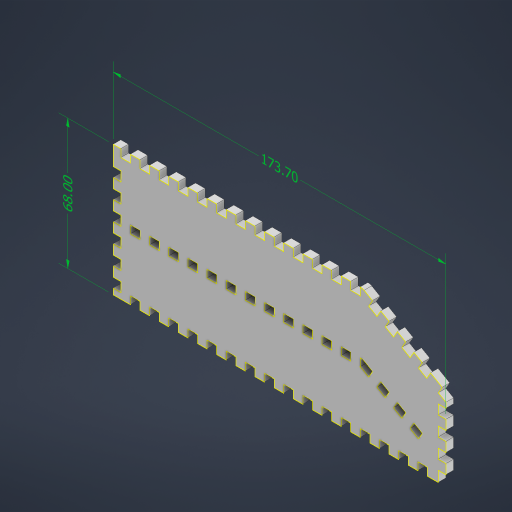
# Autodesk Inventor part: SeitenWand
Saved by Autodesk Inventor 2023 (Build 270158030, 158C)
## iProperties
Created: 2022-06-21
Part Number: SeitenWand
Material: Generic
Document SubType Name: Modeling
Designer: Simon
Density: 1 g/cm^3
Appearance: Default
Author: Simon
Autodesk Inventor part; units mm, degrees
ref_plane "YZ Plane" through (0, 0, 0) normal (1, 0, 0) x (0, 1, 0)
ref_plane "XZ Plane" through (0, 0, 0) normal (0, 1, 0) x (-1, 0, 0)
ref_plane "XY Plane" through (0, 0, 0) normal (0, 0, 1) x (1, 0, 0)
sketch "Sketch1" plane through (0, 0, 0) normal (0, 0, 1) x (1, 0, 0)
  line L0 (86, 30) -> (-86, 30)
  line L1 (-86, 30) -> (-86, -30)
  line L2 (-86, -30) -> (86, -30)
  line L3 (86, -30) -> (86, 30)
  line L4 (86, 30) -> (-86, -30) construction
  line L5 (-86, 30) -> (86, -30) construction
  line L6 (39, 30) -> (79.7032, 6.5)
  line L7 (39, 30) -> (86, 30) construction
  line L8 (79.7032, 6.5) -> (79.7032, -30)
  circle A0 centre (39, 30) radius 47
  point P0 (0, 0)
  dimension "d0" = 172
  dimension "d1" = 60
  dimension "d2" = 47
  dimension "d3" = 30
  dimension "d4" = 125
  constraints: 18 end point, 2 horizontal, 2 midpoint, 2 parallel, 2 perpendicular, 2 point on line, 1 coincident, 1 equal length, 3 other
  measures "d0" distance of L2.end L1.end
  measures "d1" distance of L1.end L0.end
  measures "d2" distance of L6.start L6.end
  measures "d3" angle of L6 L7
  measures "d4" distance of L0.end L6.start
extrude "Extrusion1" add sketch "Sketch1" along normal blind 4 contours L6 A0 L0 | L8 L2 L1 L0 A0 picked at (64.2944, 11.7777)
sketch "Sketch2" plane through (0, 0, 4) normal (0, 0, 1) x (1, 0, 0)
  line L0 (39, 30) -> (-86, 30) projected
  line L1 (-81, 30) -> (-76, 30)
  line L2 (-76, 30) -> (-76, 34)
  line L3 (-76, 34) -> (-81, 34)
  line L4 (-81, 34) -> (-81, 30)
  line L5 (-71, 30) -> (-66, 30)
  line L6 (-66, 30) -> (-66, 34)
  line L7 (-66, 34) -> (-71, 34)
  line L8 (-71, 34) -> (-71, 30)
  line L9 (-61, 30) -> (-56, 30)
  line L10 (-56, 30) -> (-56, 34)
  line L11 (-56, 34) -> (-61, 34)
  line L12 (-61, 34) -> (-61, 30)
  line L13 (-51, 30) -> (-46, 30)
  line L14 (-46, 30) -> (-46, 34)
  line L15 (-46, 34) -> (-51, 34)
  line L16 (-51, 34) -> (-51, 30)
  line L17 (-41, 30) -> (-36, 30)
  line L18 (-36, 30) -> (-36, 34)
  line L19 (-36, 34) -> (-41, 34)
  line L20 (-41, 34) -> (-41, 30)
  line L21 (-31, 30) -> (-26, 30)
  line L22 (-26, 30) -> (-26, 34)
  line L23 (-26, 34) -> (-31, 34)
  line L24 (-31, 34) -> (-31, 30)
  line L25 (-21, 30) -> (-16, 30)
  line L26 (-16, 30) -> (-16, 34)
  line L27 (-16, 34) -> (-21, 34)
  line L28 (-21, 34) -> (-21, 30)
  line L29 (-11, 30) -> (-6, 30)
  line L30 (-6, 30) -> (-6, 34)
  line L31 (-6, 34) -> (-11, 34)
  line L32 (-11, 34) -> (-11, 30)
  line L33 (-1, 30) -> (4, 30)
  line L34 (4, 30) -> (4, 34)
  line L35 (4, 34) -> (-1, 34)
  line L36 (-1, 34) -> (-1, 30)
  line L37 (9, 30) -> (14, 30)
  line L38 (14, 30) -> (14, 34)
  line L39 (14, 34) -> (9, 34)
  line L40 (9, 34) -> (9, 30)
  line L41 (19, 30) -> (24, 30)
  line L42 (24, 30) -> (24, 34)
  line L43 (24, 34) -> (19, 34)
  line L44 (19, 34) -> (19, 30)
  line L45 (29, 30) -> (34, 30)
  line L46 (34, 30) -> (34, 34)
  line L47 (34, 34) -> (29, 34)
  line L48 (29, 34) -> (29, 30)
  line L49 (79.7032, 6.5) -> (39, 30) projected
  line L50 (39, 30) -> (43.3301, 27.5)
  line L51 (43.3301, 27.5) -> (45.3301, 30.9641)
  line L52 (45.3301, 30.9641) -> (41, 33.4641)
  line L53 (41, 33.4641) -> (39, 30)
  line L54 (39, 30) -> (39, 34)
  arc A0 (41, 33.4641) -> (39, 34) centre (39, 30) ccw
  line L55 (53.9904, 25.9641) -> (49.6603, 28.4641)
  line L56 (49.6603, 28.4641) -> (47.6603, 25)
  line L57 (51.9904, 22.5) -> (53.9904, 25.9641)
  line L58 (47.6603, 25) -> (51.9904, 22.5)
  line L59 (62.6506, 20.9641) -> (58.3205, 23.4641)
  line L60 (58.3205, 23.4641) -> (56.3205, 20)
  line L61 (60.6506, 17.5) -> (62.6506, 20.9641)
  line L62 (56.3205, 20) -> (60.6506, 17.5)
  line L63 (71.3109, 15.9641) -> (66.9808, 18.4641)
  line L64 (66.9808, 18.4641) -> (64.9808, 15)
  line L65 (69.3109, 12.5) -> (71.3109, 15.9641)
  line L66 (64.9808, 15) -> (69.3109, 12.5)
  line L67 (79.9711, 10.9641) -> (75.641, 13.4641)
  line L68 (75.641, 13.4641) -> (73.641, 10)
  line L69 (77.9711, 7.5) -> (79.9711, 10.9641)
  line L70 (73.641, 10) -> (77.9711, 7.5)
  line L71 (75.641, 13.4641) -> (81.7032, 9.9641)
  line L72 (81.7032, 9.9641) -> (79.7032, 6.5)
  line L73 (-81, -2) -> (-76, -2)
  line L74 (-76, -2) -> (-76, 2)
  line L75 (-76, 2) -> (-81, 2)
  line L76 (-81, 2) -> (-81, -2)
  line L77 (-81, -2) -> (-76, 2) construction
  line L78 (-76, -2) -> (-81, 2) construction
  line L79 (-66, -2) -> (-66, 2)
  line L80 (-66, 2) -> (-71, 2)
  line L81 (-71, -2) -> (-66, -2)
  line L82 (-71, 2) -> (-71, -2)
  line L83 (-71, -2) -> (-66, 2) construction
  line L84 (-66, -2) -> (-71, 2) construction
  line L85 (-56, -2) -> (-56, 2)
  line L86 (-56, 2) -> (-61, 2)
  line L87 (-61, -2) -> (-56, -2)
  line L88 (-61, 2) -> (-61, -2)
  line L89 (-61, -2) -> (-56, 2) construction
  line L90 (-56, -2) -> (-61, 2) construction
  line L91 (-46, -2) -> (-46, 2)
  line L92 (-46, 2) -> (-51, 2)
  line L93 (-51, -2) -> (-46, -2)
  line L94 (-51, 2) -> (-51, -2)
  line L95 (-51, -2) -> (-46, 2) construction
  line L96 (-46, -2) -> (-51, 2) construction
  line L97 (-36, -2) -> (-36, 2)
  line L98 (-36, 2) -> (-41, 2)
  line L99 (-41, -2) -> (-36, -2)
  line L100 (-41, 2) -> (-41, -2)
  line L101 (-41, -2) -> (-36, 2) construction
  line L102 (-36, -2) -> (-41, 2) construction
  line L103 (-26, -2) -> (-26, 2)
  line L104 (-26, 2) -> (-31, 2)
  line L105 (-31, -2) -> (-26, -2)
  line L106 (-31, 2) -> (-31, -2)
  line L107 (-31, -2) -> (-26, 2) construction
  line L108 (-26, -2) -> (-31, 2) construction
  line L109 (-16, -2) -> (-16, 2)
  line L110 (-16, 2) -> (-21, 2)
  line L111 (-21, -2) -> (-16, -2)
  line L112 (-21, 2) -> (-21, -2)
  line L113 (-21, -2) -> (-16, 2) construction
  line L114 (-16, -2) -> (-21, 2) construction
  line L115 (-6, -2) -> (-6, 2)
  line L116 (-6, 2) -> (-11, 2)
  line L117 (-11, -2) -> (-6, -2)
  line L118 (-11, 2) -> (-11, -2)
  line L119 (-11, -2) -> (-6, 2) construction
  line L120 (-6, -2) -> (-11, 2) construction
  line L121 (4, -2) -> (4, 2)
  line L122 (4, 2) -> (-1, 2)
  line L123 (-1, -2) -> (4, -2)
  line L124 (-1, 2) -> (-1, -2)
  line L125 (-1, -2) -> (4, 2) construction
  line L126 (4, -2) -> (-1, 2) construction
  line L127 (14, -2) -> (14, 2)
  line L128 (14, 2) -> (9, 2)
  line L129 (9, -2) -> (14, -2)
  line L130 (9, 2) -> (9, -2)
  line L131 (9, -2) -> (14, 2) construction
  line L132 (14, -2) -> (9, 2) construction
  line L133 (24, -2) -> (24, 2)
  line L134 (24, 2) -> (19, 2)
  line L135 (19, -2) -> (24, -2)
  line L136 (19, 2) -> (19, -2)
  line L137 (19, -2) -> (24, 2) construction
  line L138 (24, -2) -> (19, 2) construction
  line L139 (34, -2) -> (34, 2)
  line L140 (34, 2) -> (29, 2)
  line L141 (29, -2) -> (34, -2)
  line L142 (29, 2) -> (29, -2)
  line L143 (29, -2) -> (34, 2) construction
  line L144 (34, -2) -> (29, 2) construction
  line L145 (39, -2) -> (43.3301, -4.5)
  line L146 (43.3301, -4.5) -> (45.3301, -1.0359)
  line L147 (45.3301, -1.0359) -> (41, 1.4641)
  line L148 (41, 1.4641) -> (39, -2)
  line L149 (39, -2) -> (44, -2) construction
  line L150 (39, -2) -> (39, 2)
  arc A1 (41, 1.4641) -> (39, 2) centre (39, -2) ccw
  line L151 (51.9904, -9.5) -> (53.9904, -6.0359)
  line L152 (47.6603, -7) -> (51.9904, -9.5)
  line L153 (49.6603, -3.5359) -> (47.6603, -7)
  line L154 (53.9904, -6.0359) -> (49.6603, -3.5359)
  line L155 (60.6506, -14.5) -> (62.6506, -11.0359)
  line L156 (56.3205, -12) -> (60.6506, -14.5)
  line L157 (58.3205, -8.5359) -> (56.3205, -12)
  line L158 (62.6506, -11.0359) -> (58.3205, -8.5359)
  line L159 (69.3109, -19.5) -> (71.3109, -16.0359)
  line L160 (64.9808, -17) -> (69.3109, -19.5)
  line L161 (66.9808, -13.5359) -> (64.9808, -17)
  line L162 (71.3109, -16.0359) -> (66.9808, -13.5359)
  line L163 (-86, -30) -> (79.7032, -30) projected
  line L164 (-86, -30) -> (-81, -30)
  line L165 (-81, -30) -> (-81, -34)
  line L166 (-81, -34) -> (-86, -34)
  line L167 (-86, -34) -> (-86, -30)
  line L168 (-71, -30) -> (-71, -34)
  line L169 (-76, -30) -> (-71, -30)
  line L170 (-76, -34) -> (-76, -30)
  line L171 (-71, -34) -> (-76, -34)
  line L172 (-61, -30) -> (-61, -34)
  line L173 (-66, -30) -> (-61, -30)
  line L174 (-66, -34) -> (-66, -30)
  line L175 (-61, -34) -> (-66, -34)
  line L176 (-51, -30) -> (-51, -34)
  line L177 (-56, -30) -> (-51, -30)
  line L178 (-56, -34) -> (-56, -30)
  line L179 (-51, -34) -> (-56, -34)
  line L180 (-41, -30) -> (-41, -34)
  line L181 (-46, -30) -> (-41, -30)
  line L182 (-46, -34) -> (-46, -30)
  line L183 (-41, -34) -> (-46, -34)
  line L184 (-31, -30) -> (-31, -34)
  line L185 (-36, -30) -> (-31, -30)
  line L186 (-36, -34) -> (-36, -30)
  line L187 (-31, -34) -> (-36, -34)
  line L188 (-21, -30) -> (-21, -34)
  line L189 (-26, -30) -> (-21, -30)
  line L190 (-26, -34) -> (-26, -30)
  line L191 (-21, -34) -> (-26, -34)
  line L192 (-11, -30) -> (-11, -34)
  line L193 (-16, -30) -> (-11, -30)
  line L194 (-16, -34) -> (-16, -30)
  line L195 (-11, -34) -> (-16, -34)
  line L196 (-1, -30) -> (-1, -34)
  line L197 (-6, -30) -> (-1, -30)
  line L198 (-6, -34) -> (-6, -30)
  line L199 (-1, -34) -> (-6, -34)
  line L200 (9, -30) -> (9, -34)
  line L201 (4, -30) -> (9, -30)
  line L202 (4, -34) -> (4, -30)
  line L203 (9, -34) -> (4, -34)
  line L204 (19, -30) -> (19, -34)
  line L205 (14, -30) -> (19, -30)
  line L206 (14, -34) -> (14, -30)
  line L207 (19, -34) -> (14, -34)
  line L208 (29, -30) -> (29, -34)
  line L209 (24, -30) -> (29, -30)
  line L210 (24, -34) -> (24, -30)
  line L211 (29, -34) -> (24, -34)
  line L212 (39, -30) -> (39, -34)
  line L213 (34, -30) -> (39, -30)
  line L214 (34, -34) -> (34, -30)
  line L215 (39, -34) -> (34, -34)
  line L216 (49, -30) -> (49, -34)
  line L217 (44, -30) -> (49, -30)
  line L218 (44, -34) -> (44, -30)
  line L219 (49, -34) -> (44, -34)
  line L220 (59, -30) -> (59, -34)
  line L221 (54, -30) -> (59, -30)
  line L222 (54, -34) -> (54, -30)
  line L223 (59, -34) -> (54, -34)
  line L224 (69, -30) -> (69, -34)
  line L225 (64, -30) -> (69, -30)
  line L226 (64, -34) -> (64, -30)
  line L227 (69, -34) -> (64, -34)
  line L228 (79, -30) -> (79, -34)
  line L229 (74, -30) -> (79, -30)
  line L230 (74, -34) -> (74, -30)
  line L231 (79, -34) -> (74, -34)
  line L232 (79.7032, -30) -> (79, -30)
  line L233 (79, -30) -> (79, -34)
  line L234 (79, -34) -> (79.7032, -34)
  line L235 (79.7032, -34) -> (79.7032, -30)
  point P0 (0, 0)
  point P1 (-78.5, 0)
  point P2 (-68.5, 0)
  point P3 (-58.5, 0)
  point P4 (-48.5, 0)
  point P5 (-38.5, 0)
  point P6 (-28.5, 0)
  point P7 (-18.5, 0)
  point P8 (-8.5, 0)
  point P9 (1.5, 0)
  point P10 (11.5, 0)
  point P11 (21.5, 0)
  point P12 (31.5, 0)
  dimension "d7" = 5
  dimension "d8" = 4
  dimension "d11" = 10
  dimension "d16" = 5
  dimension "d17" = 4
  dimension "d20" = 10
  dimension "d25" = 7
  dimension "d26" = 5
  dimension "d27" = 4
  dimension "d30" = 10
  dimension "d35" = 5
  dimension "d36" = 30
  dimension "d37" = 4
  dimension "d40" = 10
  dimension "d45" = 5
  dimension "d46" = 4
  dimension "d49" = 10
  constraints: 466 end point, 108 horizontal alignment, 66 parallel, 57 collinear, 6 horizontal, 6 perpendicular, 4 point on circle, 4 point on line, 2 centre point, 2 midpoint, 2 tangent, 2 vertical, 1 equal length, 179 other
  measures "d7" distance of L3.end L2.end
  measures "d8" distance of L2.end L1.end
  measures "d11" distance of L1.start L5.start
  measures "d16" distance of L49.end L50.end
  measures "d17" distance of L51.end L50.end
  measures "d20" distance of L51.end L55.start
  measures "d25" distance of L67.end L71.end
  measures "d26" distance of L75.end L74.end
  measures "d27" distance of L74.end L73.end
  measures "d30" distance of L73.end L79.start
  measures "d35" distance of L145.start L145.end
  measures "d36" angle of L145 L149
  measures "d37" distance of L146.end L145.end
  measures "d40" distance of L145.end L151.start
  measures "d45" distance of L165.end L166.end
  measures "d46" distance of L164.end L165.end
  measures "d49" distance of L164.end L168.start
extrude "Extrusion2" add sketch "Sketch2" against normal blind 4 contours L0 L48 L47 L46 | L0 L44 L43 L42 | L0 L40 L39 L38 | L0 L36 L35 L34 | L0 L32 L31 L30 | L0 L28 L27 L26 | L0 L24 L23 L22 | L0 L20 L19 L18 | L0 L16 L15 L14 | L0 L12 L11 L10 | L0 L8 L7 L6 | L0 L4 L3 L2 | L49 L69 L71 L72 | L49 L68 L67 L69 | L49 L64 L63 L65 | L49 L60 L59 L61 | L49 L56 L55 L57 | L49 L53 L52 L51 | L54 A0 L53 | L163 L165 L166 L167 | L163 L168 L171 L170 | L163 L172 L175 L174 | L163 L176 L179 L178 | L163 L180 L183 L182 | L163 L184 L187 L186 | L163 L188 L191 L190 | L163 L192 L195 L194 | L163 L196 L199 L198 | L163 L200 L203 L202 | L163 L204 L207 L206 | L163 L208 L211 L210 | L163 L212 L215 L214 | L163 L216 L219 L218 | L163 L220 L223 L222 | L163 L224 L227 L226 | L163 L228 L231 L230 | L163 L235 L234 L228
extrude "Extrusion3" cut sketch "Sketch2" against normal blind 4 contours L76 L75 L74 L73 | L81 L82 L80 L79 | L87 L88 L86 L85 | L93 L94 L92 L91 | L99 L100 L98 L97 | L105 L106 L104 L103 | L111 L112 L110 L109 | L117 L118 L116 L115 | L123 L124 L122 L121 | L129 L130 L128 L127 | L135 L136 L134 L133 | L141 L142 L140 L139 | L148 L147 L146 L145 | L150 A1 L148 | L152 L153 L154 L151 | L156 L157 L158 L155 | L160 L161 L162 L159
sketch "Sketch3" plane through (0, 0, 4) normal (0, 0, 1) x (1, 0, 0)
  line L0 (-86, 34) -> (-90, 34)
  line L1 (-90, 34) -> (-90, 24)
  line L2 (-90, 24) -> (-86, 24)
  line L3 (-86, 24) -> (-86, 34)
  line L4 (-86, 30) -> (-86, -34) projected
  line L5 (-86, 19) -> (-90, 19)
  line L6 (-90, 19) -> (-90, 14)
  line L7 (-90, 14) -> (-86, 14)
  line L8 (-86, 14) -> (-86, 19)
  line L9 (-86, 9) -> (-90, 9)
  line L10 (-90, 9) -> (-90, 4)
  line L11 (-90, 4) -> (-86, 4)
  line L12 (-86, 4) -> (-86, 9)
  line L13 (-86, -1) -> (-90, -1)
  line L14 (-90, -1) -> (-90, -6)
  line L15 (-90, -6) -> (-86, -6)
  line L16 (-86, -6) -> (-86, -1)
  line L17 (-86, -11) -> (-90, -11)
  line L18 (-90, -11) -> (-90, -16)
  line L19 (-90, -16) -> (-86, -16)
  line L20 (-86, -16) -> (-86, -11)
  line L21 (-86, -21) -> (-90, -21)
  line L22 (-90, -21) -> (-90, -26)
  line L23 (-90, -26) -> (-86, -26)
  line L24 (-86, -26) -> (-86, -21)
  line L25 (-86, -31) -> (-90, -31)
  line L26 (-90, -31) -> (-90, -36)
  line L27 (-90, -36) -> (-86, -36)
  line L28 (-86, -36) -> (-86, -31)
  line L29 (-86, -34) -> (-81, -34) projected
  line L30 (-86, -34) -> (-90, -34)
  point P0 (0, 0)
  dimension "d58" = 4
  dimension "d59" = 10
  dimension "d60" = 4
  dimension "d61" = 5
  dimension "d64" = 10
  constraints: 58 end point, 4 parallel, 3 perpendicular, 2 horizontal, 2 point on line, 1 vertical, 40 other
  measures "d58" distance of L2.end L1.end
  measures "d59" distance of L1.end L0.end
  measures "d60" distance of L7.end L6.end
  measures "d61" distance of L6.end L5.end
  measures "d64" distance of L5.start L9.start
extrude "Extrusion4" add sketch "Sketch3" against normal blind 4 contours L3 L2 L1 L0 | L4 L7 L6 L5 | L4 L11 L10 L9 | L4 L15 L14 L13 | L4 L19 L18 L17 | L4 L23 L22 L21 | L4 L30 L26 L25
sketch "Sketch4" plane through (0, 0, 4) normal (0, 0, 1) x (1, 0, 0)
  line L0 (81.7032, 9.9641) -> (79.7032, 6.5) projected
  line L1 (79.7032, 6.5) -> (81.7032, 9.9641)
  line L2 (81.7032, 9.9641) -> (86.0333, 7.4641)
  line L3 (86.0333, 7.4641) -> (84.0333, 4)
  line L4 (84.0333, 4) -> (79.7032, 6.5)
  line L5 (83.7032, 6.5) -> (83.7032, 1.5)
  line L6 (83.7032, 1.5) -> (79.7032, 1.5)
  line L7 (79.7032, 6.5) -> (79.7032, -34) projected
  line L8 (79.7032, 1.5) -> (79.7032, 6.5)
  line L9 (79.7032, 6.5) -> (84.0333, 4)
  line L10 (79.7032, -3.5) -> (83.7032, -3.5)
  line L11 (83.7032, -3.5) -> (83.7032, -8.5)
  line L12 (83.7032, -8.5) -> (79.7032, -8.5)
  line L13 (79.7032, -8.5) -> (79.7032, -3.5)
  line L14 (79.7032, -13.5) -> (83.7032, -13.5)
  line L15 (83.7032, -13.5) -> (83.7032, -18.5)
  line L16 (83.7032, -18.5) -> (79.7032, -18.5)
  line L17 (79.7032, -18.5) -> (79.7032, -13.5)
  line L18 (79.7032, -23.5) -> (83.7032, -23.5)
  line L19 (83.7032, -23.5) -> (83.7032, -28.5)
  line L20 (83.7032, -28.5) -> (79.7032, -28.5)
  line L21 (79.7032, -28.5) -> (79.7032, -23.5)
  line L22 (79.7032, 6.5) -> (83.7032, 4.1906)
  line L23 (83.7032, 1.5) -> (83.7032, 4.1906)
  point P0 (0, 0)
  dimension "d71" = 5
  dimension "d72" = 5
  dimension "d73" = 4
  dimension "d74" = 4
  dimension "d75" = 5
  dimension "d78" = 10
  constraints: 44 end point, 4 collinear, 4 parallel, 3 perpendicular, 3 point on line, 2 vertical, 1 horizontal, 15 other
  measures "d71" distance of L0.start L2.end
  measures "d72" distance of L5.start L5.end
  measures "d73" distance of L5.end L6.end
  measures "d74" distance of L11.end L12.end
  measures "d75" distance of L10.end L11.end
  measures "d78" distance of L10.start L14.start
extrude "Extrusion5" add sketch "Sketch4" against normal blind 4 contours L4 L5 L6 L7 | L10 L11 L12 L7 | L14 L15 L16 L7 | L18 L19 L20 L7
sketch "Sketch5" plane through (0, 0, 4) normal (0, 0, 1) x (1, 0, 0)
  line L0 (-11, -2) -> (-11, 2) projected
  line L1 (-11, 2) -> (-6, 2) projected
  line L2 (-6, 2) -> (-6, -2) projected
  line L3 (-6, -2) -> (-11, -2) projected
  line L4 (-51, -2) -> (-51, 2) projected
  line L5 (-51, 2) -> (-46, 2) projected
  line L6 (-46, 2) -> (-46, -2) projected
  line L7 (-46, -2) -> (-51, -2) projected
  line L8 (47.6603, -7) -> (49.6603, -3.5359) projected
  line L9 (49.6603, -3.5359) -> (53.9904, -6.0359) projected
  line L10 (53.9904, -6.0359) -> (51.9904, -9.5) projected
  line L11 (51.9904, -9.5) -> (47.6603, -7) projected
  line L12 (9, -2) -> (9, 2) projected
  line L13 (9, 2) -> (14, 2) projected
  line L14 (14, 2) -> (14, -2) projected
  line L15 (14, -2) -> (9, -2) projected
  line L16 (19, -2) -> (19, 2) projected
  line L17 (19, 2) -> (24, 2) projected
  line L18 (24, 2) -> (24, -2) projected
  line L19 (24, -2) -> (19, -2) projected
  line L20 (56.3205, -12) -> (58.3205, -8.5359) projected
  line L21 (58.3205, -8.5359) -> (62.6506, -11.0359) projected
  line L22 (62.6506, -11.0359) -> (60.6506, -14.5) projected
  line L23 (60.6506, -14.5) -> (56.3205, -12) projected
  line L24 (-41, -2) -> (-41, 2) projected
  line L25 (-41, 2) -> (-36, 2) projected
  line L26 (-36, 2) -> (-36, -2) projected
  line L27 (-36, -2) -> (-41, -2) projected
  line L28 (-71, -2) -> (-71, 2) projected
  line L29 (-71, 2) -> (-66, 2) projected
  line L30 (-66, 2) -> (-66, -2) projected
  line L31 (-66, -2) -> (-71, -2) projected
  line L32 (-21, -2) -> (-21, 2) projected
  line L33 (-21, 2) -> (-16, 2) projected
  line L34 (-16, 2) -> (-16, -2) projected
  line L35 (-16, -2) -> (-21, -2) projected
  line L36 (-61, -2) -> (-61, 2) projected
  line L37 (-61, 2) -> (-56, 2) projected
  line L38 (-56, 2) -> (-56, -2) projected
  line L39 (-56, -2) -> (-61, -2) projected
  line L40 (43.3301, -4.5) -> (39, -2) projected
  line L41 (39, -2) -> (39, 2) projected
  arc A0 (41, 1.4641) -> (39, 2) centre (39, -2) ccw projected
  line L42 (41, 1.4641) -> (45.3301, -1.0359) projected
  line L43 (45.3301, -1.0359) -> (43.3301, -4.5) projected
  line L44 (-1, -2) -> (-1, 2) projected
  line L45 (-1, 2) -> (4, 2) projected
  line L46 (4, 2) -> (4, -2) projected
  line L47 (4, -2) -> (-1, -2) projected
  line L48 (29, -2) -> (29, 2) projected
  line L49 (29, 2) -> (34, 2) projected
  line L50 (34, 2) -> (34, -2) projected
  line L51 (34, -2) -> (29, -2) projected
  line L52 (64.9808, -17) -> (66.9808, -13.5359) projected
  line L53 (66.9808, -13.5359) -> (71.3109, -16.0359) projected
  line L54 (71.3109, -16.0359) -> (69.3109, -19.5) projected
  line L55 (69.3109, -19.5) -> (64.9808, -17) projected
  line L56 (-31, -2) -> (-31, 2) projected
  line L57 (-31, 2) -> (-26, 2) projected
  line L58 (-26, 2) -> (-26, -2) projected
  line L59 (-26, -2) -> (-31, -2) projected
  line L60 (-81, 2) -> (-76, 2) projected
  line L61 (-76, 2) -> (-76, -2) projected
  line L62 (-76, -2) -> (-81, -2) projected
  line L63 (-81, -2) -> (-81, 2) projected
  line L64 (-81, -30) -> (-76, -30) projected
  line L65 (-76, -30) -> (-76, -34) projected
  line L66 (-76, -34) -> (-71, -34) projected
  line L67 (-71, -34) -> (-71, -30) projected
  line L68 (-71, -30) -> (-66, -30) projected
  line L69 (-66, -30) -> (-66, -34) projected
  line L70 (-66, -34) -> (-61, -34) projected
  line L71 (-61, -34) -> (-61, -30) projected
  line L72 (-61, -30) -> (-56, -30) projected
  line L73 (-56, -30) -> (-56, -34) projected
  line L74 (-56, -34) -> (-51, -34) projected
  line L75 (-51, -34) -> (-51, -30) projected
  line L76 (-51, -30) -> (-46, -30) projected
  line L77 (-46, -30) -> (-46, -34) projected
  line L78 (-46, -34) -> (-41, -34) projected
  line L79 (-41, -34) -> (-41, -30) projected
  line L80 (-41, -30) -> (-36, -30) projected
  line L81 (-36, -30) -> (-36, -34) projected
  line L82 (-36, -34) -> (-31, -34) projected
  line L83 (-31, -34) -> (-31, -30) projected
  line L84 (-31, -30) -> (-26, -30) projected
  line L85 (-26, -30) -> (-26, -34) projected
  line L86 (-26, -34) -> (-21, -34) projected
  line L87 (-21, -34) -> (-21, -30) projected
  line L88 (-21, -30) -> (-16, -30) projected
  line L89 (-16, -30) -> (-16, -34) projected
  line L90 (-16, -34) -> (-11, -34) projected
  line L91 (-11, -34) -> (-11, -30) projected
  line L92 (-11, -30) -> (-6, -30) projected
  line L93 (-6, -30) -> (-6, -34) projected
  line L94 (-6, -34) -> (-1, -34) projected
  line L95 (-1, -34) -> (-1, -30) projected
  line L96 (-1, -30) -> (4, -30) projected
  line L97 (4, -30) -> (4, -34) projected
  line L98 (4, -34) -> (9, -34) projected
  line L99 (9, -34) -> (9, -30) projected
  line L100 (9, -30) -> (14, -30) projected
  line L101 (14, -30) -> (14, -34) projected
  line L102 (14, -34) -> (19, -34) projected
  line L103 (19, -34) -> (19, -30) projected
  line L104 (19, -30) -> (24, -30) projected
  line L105 (24, -30) -> (24, -34) projected
  line L106 (24, -34) -> (29, -34) projected
  line L107 (29, -34) -> (29, -30) projected
  line L108 (29, -30) -> (34, -30) projected
  line L109 (34, -30) -> (34, -34) projected
  line L110 (34, -34) -> (39, -34) projected
  line L111 (39, -34) -> (39, -30) projected
  line L112 (39, -30) -> (44, -30) projected
  line L113 (44, -30) -> (44, -34) projected
  line L114 (44, -34) -> (49, -34) projected
  line L115 (49, -34) -> (49, -30) projected
  line L116 (49, -30) -> (54, -30) projected
  line L117 (54, -30) -> (54, -34) projected
  line L118 (54, -34) -> (59, -34) projected
  line L119 (59, -34) -> (59, -30) projected
  line L120 (59, -30) -> (64, -30) projected
  line L121 (64, -30) -> (64, -34) projected
  line L122 (64, -34) -> (69, -34) projected
  line L123 (69, -34) -> (69, -30) projected
  line L124 (69, -30) -> (74, -30) projected
  line L125 (74, -30) -> (74, -34) projected
  line L126 (74, -34) -> (79.7032, -34) projected
  line L127 (79.7032, -34) -> (79.7032, -28.5) projected
  line L128 (79.7032, -28.5) -> (83.7032, -28.5) projected
  line L129 (83.7032, -28.5) -> (83.7032, -23.5) projected
  line L130 (83.7032, -23.5) -> (79.7032, -23.5) projected
  line L131 (79.7032, -23.5) -> (79.7032, -18.5) projected
  line L132 (79.7032, -18.5) -> (83.7032, -18.5) projected
  line L133 (83.7032, -18.5) -> (83.7032, -13.5) projected
  line L134 (83.7032, -13.5) -> (79.7032, -13.5) projected
  line L135 (79.7032, -13.5) -> (79.7032, -8.5) projected
  line L136 (79.7032, -8.5) -> (83.7032, -8.5) projected
  line L137 (83.7032, -8.5) -> (83.7032, -3.5) projected
  line L138 (83.7032, -3.5) -> (79.7032, -3.5) projected
  line L139 (79.7032, -3.5) -> (79.7032, 1.5) projected
  line L140 (79.7032, 1.5) -> (83.7032, 1.5) projected
  line L141 (83.7032, 1.5) -> (83.7032, 4.1906) projected
  line L142 (83.7032, 4.1906) -> (79.7032, 6.5) projected
  line L143 (79.7032, 6.5) -> (81.7032, 9.9641) projected
  line L144 (81.7032, 9.9641) -> (75.641, 13.4641) projected
  line L145 (75.641, 13.4641) -> (73.641, 10) projected
  line L146 (73.641, 10) -> (69.3109, 12.5) projected
  line L147 (69.3109, 12.5) -> (71.3109, 15.9641) projected
  line L148 (71.3109, 15.9641) -> (66.9808, 18.4641) projected
  line L149 (66.9808, 18.4641) -> (64.9808, 15) projected
  line L150 (64.9808, 15) -> (60.6506, 17.5) projected
  line L151 (60.6506, 17.5) -> (62.6506, 20.9641) projected
  line L152 (62.6506, 20.9641) -> (58.3205, 23.4641) projected
  line L153 (58.3205, 23.4641) -> (56.3205, 20) projected
  line L154 (56.3205, 20) -> (51.9904, 22.5) projected
  line L155 (51.9904, 22.5) -> (53.9904, 25.9641) projected
  line L156 (53.9904, 25.9641) -> (49.6603, 28.4641) projected
  line L157 (49.6603, 28.4641) -> (47.6603, 25) projected
  line L158 (47.6603, 25) -> (43.3301, 27.5) projected
  line L159 (43.3301, 27.5) -> (45.3301, 30.9641) projected
  line L160 (45.3301, 30.9641) -> (41, 33.4641) projected
  arc A1 (41, 33.4641) -> (39, 34) centre (39, 30) ccw projected
  line L161 (39, 34) -> (39, 30) projected
  line L162 (39, 30) -> (34, 30) projected
  line L163 (34, 30) -> (34, 34) projected
  line L164 (34, 34) -> (29, 34) projected
  line L165 (29, 34) -> (29, 30) projected
  line L166 (29, 30) -> (24, 30) projected
  line L167 (24, 30) -> (24, 34) projected
  line L168 (24, 34) -> (19, 34) projected
  line L169 (19, 34) -> (19, 30) projected
  line L170 (19, 30) -> (14, 30) projected
  line L171 (14, 30) -> (14, 34) projected
  line L172 (14, 34) -> (9, 34) projected
  line L173 (9, 34) -> (9, 30) projected
  line L174 (9, 30) -> (4, 30) projected
  line L175 (4, 30) -> (4, 34) projected
  line L176 (4, 34) -> (-1, 34) projected
  line L177 (-1, 34) -> (-1, 30) projected
  line L178 (-1, 30) -> (-6, 30) projected
  line L179 (-6, 30) -> (-6, 34) projected
  line L180 (-6, 34) -> (-11, 34) projected
  line L181 (-11, 34) -> (-11, 30) projected
  line L182 (-11, 30) -> (-16, 30) projected
  line L183 (-16, 30) -> (-16, 34) projected
  line L184 (-16, 34) -> (-21, 34) projected
  line L185 (-21, 34) -> (-21, 30) projected
  line L186 (-21, 30) -> (-26, 30) projected
  line L187 (-26, 30) -> (-26, 34) projected
  line L188 (-26, 34) -> (-31, 34) projected
  line L189 (-31, 34) -> (-31, 30) projected
  line L190 (-31, 30) -> (-36, 30) projected
  line L191 (-36, 30) -> (-36, 34) projected
  line L192 (-36, 34) -> (-41, 34) projected
  line L193 (-41, 34) -> (-41, 30) projected
  line L194 (-41, 30) -> (-46, 30) projected
  line L195 (-46, 30) -> (-46, 34) projected
  line L196 (-46, 34) -> (-51, 34) projected
  line L197 (-51, 34) -> (-51, 30) projected
  line L198 (-51, 30) -> (-56, 30) projected
  line L199 (-56, 30) -> (-56, 34) projected
  line L200 (-56, 34) -> (-61, 34) projected
  line L201 (-61, 34) -> (-61, 30) projected
  line L202 (-61, 30) -> (-66, 30) projected
  line L203 (-66, 30) -> (-66, 34) projected
  line L204 (-66, 34) -> (-71, 34) projected
  line L205 (-71, 34) -> (-71, 30) projected
  line L206 (-71, 30) -> (-76, 30) projected
  line L207 (-76, 30) -> (-76, 34) projected
  line L208 (-76, 34) -> (-81, 34) projected
  line L209 (-81, 34) -> (-81, 30) projected
  line L210 (-81, 30) -> (-86, 30) projected
  line L211 (-86, 30) -> (-86, 34) projected
  line L212 (-86, 34) -> (-90, 34) projected
  line L213 (-90, 34) -> (-90, 24) projected
  line L214 (-90, 24) -> (-86, 24) projected
  line L215 (-86, 24) -> (-86, 19) projected
  line L216 (-86, 19) -> (-90, 19) projected
  line L217 (-90, 19) -> (-90, 14) projected
  line L218 (-90, 14) -> (-86, 14) projected
  line L219 (-86, 14) -> (-86, 9) projected
  line L220 (-86, 9) -> (-90, 9) projected
  line L221 (-90, 9) -> (-90, 4) projected
  line L222 (-90, 4) -> (-86, 4) projected
  line L223 (-86, 4) -> (-86, -1) projected
  line L224 (-86, -1) -> (-90, -1) projected
  line L225 (-90, -1) -> (-90, -6) projected
  line L226 (-90, -6) -> (-86, -6) projected
  line L227 (-86, -6) -> (-86, -11) projected
  line L228 (-86, -11) -> (-90, -11) projected
  line L229 (-90, -11) -> (-90, -16) projected
  line L230 (-90, -16) -> (-86, -16) projected
  line L231 (-86, -16) -> (-86, -21) projected
  line L232 (-86, -21) -> (-90, -21) projected
  line L233 (-90, -21) -> (-90, -26) projected
  line L234 (-90, -26) -> (-86, -26) projected
  line L235 (-86, -26) -> (-86, -31) projected
  line L236 (-86, -31) -> (-90, -31) projected
  line L237 (-90, -31) -> (-90, -34) projected
  line L238 (-90, -34) -> (-81, -34) projected
  line L239 (-81, -34) -> (-81, -30) projected
  point P0 (0, 0)
body "Solid1"
